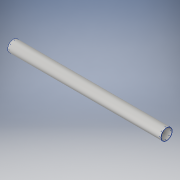
# Autodesk Inventor part: motor_casing
Saved by Autodesk Inventor 2017 SP1 (Build 210196100, 196)
## iProperties
Created: 2016-10-29
Part Number: motor_casing
Material: Aluminum 6061
Document SubType Name: Modeling
Designer: cflannery
Density: 2.7 g/cm^3
Appearance: Aluminum - Flat
Author: cflannery
Autodesk Inventor part; units mm, degrees
ref_plane "YZ Plane" through (0, 0, 0) normal (1, 0, 0) x (0, 1, 0)
ref_plane "XZ Plane" through (0, 0, 0) normal (0, 1, 0) x (-1, 0, 0)
sketch "Sketch1" plane through (0, 0, 0) normal (1, 0, 0) x (0, 1, 0)
  circle A0 centre (0, 0) radius 101.6
  circle A1 centre (0, 0) radius 95.25
  dimension "d0" = 190.5
  dimension "d1" = 203.2
  constraints: 2 centre point, 2 coincident
  measures "d0" diameter of A1
  measures "d1" diameter of A0
extrude "Extrusion1" add sketch "Sketch1" along normal blind 2743.2
ref_plane "Work Plane1" through (0, 0, 101.6) normal (0, 0, 1) x (1, 0, 0)
sketch "Sketch2" plane through (0, 0, 101.6) normal (0, 0, 1) x (1, 0, 0)
  line L0 (2743.2, -101.6) -> (2743.2, 101.6) projected
  point P0 (0, 0)
  point P1 (2717.8, 0)
  dimension "d4" = 25.4
  constraints: 1 horizontal alignment
  measures "d4" distance from line of L0 point (2717.8, 0)
hole "Hole1" at (2717.8, 0, 101.6) direction (0, 0, -1) diameter 6.35 depth 25.4 tip angle 118
pattern_circular "Circular Pattern1" count 8 over 360 about axis through (0, 0, 0) along (1, 0, 0) of "Hole1"
sketch "Sketch3" plane through (0, 0, 101.6) normal (0, 0, 1) x (1, 0, 0)
  point P0 (0, 0)
  point P1 (25.4, 0)
  dimension "d15" = 25.4
  measures "d15" distance of point (0, 0) point (25.4, 0)
hole "Hole2" at (25.4, 0, 101.6) direction (0, 0, -1) diameter 6.35 depth 25.4 tip angle 118
pattern_circular "Circular Pattern2" count 8 over 360 about axis through (0, 0, 0) along (1, 0, 0) of "Hole2"
body "Solid1"
